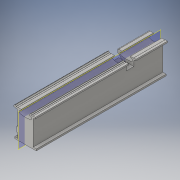
# Autodesk Inventor part: BED
Saved by Autodesk Inventor 2016 (Build 200138000, 138)
## iProperties
Created: 2017-02-14
Part Number: BED
Material: Generic
Document SubType Name: Modeling
Designer: M228540
Density: 1 g/cm^3
Appearance: Default
Author: M228540
Autodesk Inventor part; units mm, degrees
ref_plane "YZ Plane" through (0, 0, 0) normal (1, 0, 0) x (0, 1, 0)
ref_plane "XZ Plane" through (0, 0, 0) normal (0, 1, 0) x (-1, 0, 0)
ref_plane "XY Plane" through (0, 0, 0) normal (0, 0, 1) x (1, 0, 0)
sketch "Sketch1" plane through (0, 0, 0) normal (0, 0, 1) x (1, 0, 0)
  line L0 (11.5932, 5.302) -> (2.0669, 10.802)
  line L1 (11.5932, 5.302) -> (22.5932, 5.302) construction
  line L2 (2.0669, 10.802) -> (-7.9331, 10.802)
  line L3 (-7.9331, 10.802) -> (-7.9331, 22.502)
  line L4 (-7.9331, 22.502) -> (0.166, 32.1541)
  line L5 (0.166, 32.1541) -> (3.966, 32.1541)
  line L6 (3.966, 32.1541) -> (11.7797, 25.5977)
  line L7 (11.7797, 25.5977) -> (11.7797, 22.3977)
  line L8 (11.7797, 22.3977) -> (27.8797, 22.3977)
  line L9 (27.8797, 22.3977) -> (27.8797, 24.3977)
  line L10 (27.8797, 24.3977) -> (53.0797, 24.3977)
  line L11 (53.0797, 24.3977) -> (53.0797, 8.6977)
  line L12 (53.0797, 8.6977) -> (38.3797, 8.6977)
  line L13 (38.3797, 8.6977) -> (38.3797, 0.6977) construction
  line L14 (38.3797, 0.6977) -> (33.7609, 0.6977) construction
  line L15 (38.3797, 8.6977) -> (33.7609, 0.6977)
  line L16 (38.3797, 8.6977) -> (62.019, 8.6977) construction
  line L17 (33.7609, 0.6977) -> (33.7609, -3.3023) construction
  arc A0 (33.7609, 0.6977) -> (29.7609, -3.3023) centre (33.7609, -3.3023) ccw
  line L18 (29.7609, -3.3023) -> (29.7609, -65.3023)
  line L19 (29.7609, -65.3023) -> (29.7609, -269.3023)
  line L20 (-7.9331, 10.802) -> (84.2692, 10.802) construction
  line L21 (-100.1287, 11.7042) -> (-99.7212, 24.3977)
  line L22 (-99.7212, 24.3977) -> (-135.9212, 24.3977)
  line L23 (-99.7212, 24.3977) -> (-63.5212, 24.3977) construction
  line L24 (-135.9212, 24.3977) -> (-135.9212, 22.3977)
  line L25 (-135.9212, 22.3977) -> (-154.9212, 22.3977)
  line L26 (-154.9212, 22.3977) -> (-154.9212, 24.3977)
  line L27 (-154.9212, 24.3977) -> (-163.406, 34.5095)
  line L28 (-163.406, 34.5095) -> (-168.006, 34.5095)
  line L29 (-168.006, 34.5095) -> (-180.2627, 24.2249)
  line L30 (-180.2627, 24.2249) -> (-180.2627, 10.2249)
  line L31 (-180.2627, 10.2249) -> (-166.2627, 10.2249)
  line L32 (-166.2627, 10.2249) -> (-166.2627, 7.2249) construction
  line L33 (-166.2627, 7.2249) -> (-164.5307, 7.2249) construction
  line L34 (-166.2627, 10.2249) -> (-164.5307, 7.2249)
  line L35 (-166.2627, 10.2249) -> (-161.6857, 10.2249) construction
  line L36 (-164.5307, 7.2249) -> (-146.1307, 7.2249)
  line L37 (-146.1307, 7.2249) -> (-146.1307, -15.2751)
  line L38 (-146.1307, -15.2751) -> (-146.1307, -24.7751) construction
  arc A1 (-136.6307, -24.7751) -> (-146.1307, -15.2751) centre (-146.1307, -24.7751) ccw
  line L39 (-136.6307, -24.7751) -> (-136.6307, -160.7751)
  line L40 (-136.6307, -24.7751) -> (-0.6307, -24.7751) construction
  line L41 (-136.6307, -160.7751) -> (-149.6307, -160.7751)
  line L42 (-149.6307, -160.7751) -> (-149.6307, -216.2751)
  line L43 (-149.6307, -216.2751) -> (-136.6307, -216.2751)
  line L44 (-136.6307, -216.2751) -> (-136.6307, -269.3023)
  line L45 (-136.6307, -24.7751) -> (-146.1307, -24.7751) construction
  line L46 (29.7609, -3.3023) -> (33.7609, -3.3023) construction
  line L47 (-136.6307, -269.3023) -> (-171.6307, -269.3023)
  line L48 (-136.6307, -269.3023) -> (-101.6307, -269.3023) construction
  line L49 (-171.6307, -269.3023) -> (-171.6307, -287.3023)
  line L50 (29.7609, -269.3023) -> (64.7609, -269.3023)
  line L51 (29.7609, -269.3023) -> (64.7609, -269.3023) construction
  line L52 (64.7609, -269.3023) -> (64.7609, -287.3023)
  line L53 (64.7609, -287.3023) -> (-171.6307, -287.3023)
  line L54 (-100.1287, 11.7042) -> (-110.7287, 11.7042)
  line L55 (-100.1287, 11.7042) -> (-89.5287, 11.7042) construction
  line L56 (-110.7287, 11.7042) -> (-114.7287, 4.776)
  line L57 (-114.7287, 4.776) -> (-119.5691, 2.2026) construction
  line L58 (-119.5691, 2.2026) -> (-124.3726, -3.2958) construction
  line L59 (-124.3726, -3.2958) -> (-125.2569, -13.4593) construction
  line L60 (-125.2569, -13.4593) -> (-112.7287, -23.6091) construction
  line L61 (-112.7287, -23.6091) -> (-52.4666, -29.8459) construction
  line L62 (-52.4666, -29.8459) -> (0.1681, -24.7751) construction
  line L63 (0.1681, -24.7751) -> (13.3927, -18.0576) construction
  line L64 (13.3927, -18.0576) -> (19.8318, -6.9438) construction
  line L65 (19.8318, -6.9438) -> (14.7088, 3.5032) construction
  line L66 (14.7088, 3.5032) -> (11.5932, 5.302) construction
  spline S0 degree 4 poles (-114.7287, 4.776) (-119.5691, 2.2026) (-124.3726, -3.2958) (-125.2569, -13.4593) (-112.7287, -23.6091) (-52.4666, -29.8459) (0.1681, -24.7751) (13.3927, -18.0576) (19.8318, -6.9438) (14.7088, 3.5032) (11.5932, 5.302) knots 0 0 0 0 0 1 2 3 4 5 6 7 7 7 7 7
  point P0 (0, 0)
  dimension "d0" = 11
  dimension "d1" = 150
  dimension "d2" = 10
  dimension "d3" = 11.7
  dimension "d4" = 12.6
  dimension "d5" = 140
  dimension "d6" = 3.8
  dimension "d7" = 10.2
  dimension "d8" = 140
  dimension "d9" = 3.2
  dimension "d10" = 16.1
  dimension "d11" = 2
  dimension "d12" = 25.2
  dimension "d13" = 15.7
  dimension "d14" = 14.7
  dimension "d15" = 8
  dimension "d16" = 120
  dimension "d17" = 4
  dimension "d18" = 62
  dimension "d19" = 204
  dimension "d22" = 92.2
  dimension "d24" = 12.7
  dimension "d25" = 36.2
  dimension "d26" = 180
  dimension "d27" = 2
  dimension "d28" = 19
  dimension "d29" = 2
  dimension "d30" = 13.2
  dimension "d31" = 140
  dimension "d32" = 4.6
  dimension "d33" = 16
  dimension "d34" = 140
  dimension "d35" = 14
  dimension "d36" = 14
  dimension "d37" = 90
  dimension "d38" = 3
  dimension "d39" = 60
  dimension "d40" = 18.4
  dimension "d41" = 22.5
  dimension "d42" = 9.5
  dimension "d43" = 136
  dimension "d44" = 90
  dimension "d45" = 13
  dimension "d46" = 55.5
  dimension "d47" = 90
  dimension "d50" = 90
  dimension "d51" = 35
  dimension "d52" = 180
  dimension "d53" = 18
  dimension "d54" = 90
  dimension "d55" = 35
  dimension "d57" = 18
  dimension "d58" = 10.6
  dimension "d59" = 180
  dimension "d60" = 8
  dimension "d61" = 120
  dimension "d62" = 62
  constraints: 114 end point, 20 horizontal, 19 perpendicular, 6 equal length, 6 vertical, 4 point on circle, 4 point on line, 2 centre point, 2 coincident, 2 parallel, 1 collinear, 3 other
  measures "d0" distance of L0.start L0.end
  measures "d1" angle of L1 L0
  measures "d2" distance of L0.end L2.end
  measures "d3" distance of L2.end L3.end
  measures "d4" distance of L3.end L4.end
  measures "d5" angle of L3 L4
  measures "d6" distance of L4.end L5.end
  measures "d7" distance of L5.end L6.end
  measures "d8" angle of L5 L6
  measures "d9" distance of L6.end L7.end
  measures "d10" distance of L7.end L8.end
  measures "d11" distance of L8.end L9.end
  measures "d12" distance of L9.end L10.end
  measures "d13" distance of L10.end L11.end
  measures "d14" distance of L11.end L12.end
  measures "d15" distance of L12.end L13.end
  measures "d16" angle of L15 L16
  measures "d17" distance of L14.end L17.end
  measures "d18" distance of L18.start L18.end
  measures "d19" distance of L18.end L19.end
  measures "d22" distance of L2.end L21.start
  measures "d24" distance of L21.start L21.end
  measures "d25" distance of L21.end L22.end
  measures "d26" angle of L22 L23
  measures "d27" distance of L22.end L24.end
  measures "d28" distance of L24.end L25.end
  measures "d29" distance of L25.end L26.end
  measures "d30" distance of L26.end L27.end
  measures "d31" angle of L27 L26
  measures "d32" distance of L27.end L28.end
  measures "d33" distance of L28.end L29.end
  measures "d34" angle of L29 L28
  measures "d35" distance of L29.end L30.end
  measures "d36" distance of L30.end L31.end
  measures "d37" angle of L31 L30
  measures "d38" distance of L31.end L32.end
  measures "d39" angle of L34 L35
  measures "d40" distance of L33.end L36.end
  measures "d41" distance of L36.end L37.end
  measures "d42" distance of L37.end L38.end
  measures "d43" distance of L39.start L39.end
  measures "d44" angle of L39 L40
  measures "d45" distance of L39.end L41.end
  measures "d46" distance of L41.end L42.end
  measures "d47" angle of L42 L41
  measures "d50" angle of L43 L44
  measures "d51" distance of L44.end L47.end
  measures "d52" angle of L47 L48
  measures "d53" distance of L47.end L49.end
  measures "d54" angle of L49 L47
  measures "d55" distance of L19.end L50.end
  measures "d57" distance of L50.end L52.end
  measures "d58" distance of L21.start L54.end
  measures "d59" angle of L54 L55
  measures "d60" distance of L54.end L56.end
  measures "d61" angle of L56 L54
  measures "d62" distance from line of L5 L61.end
extrude "Extrusion1" add sketch "Sketch1" against normal blind 1420
chamfer "Chamfer1" distance 9 angle 45 2 edges at (-136.6307, -160.7751, -710) (-136.6307, -216.2751, -710)
ref_plane "Work Plane3" through (-63.5915, 24.2249, -1420) normal (-1, 0, 0) x (0, 0, 1)
sketch "Sketch2" plane through (-63.5915, 24.2249, -1420) normal (-1, 0, 0) x (0, 0, 1)
  line L0 (1420, 7.9293) -> (0, 7.9293) projected
  line L1 (400, 7.9293) -> (400, -79.7707)
  line L2 (400, -79.7707) -> (318, -79.7707)
  line L3 (318, -79.7707) -> (318, 139.9542)
  line L4 (1420, -27.5272) -> (0, -27.5272) projected
  line L5 (318, 139.9542) -> (400, 139.9542)
  line L6 (400, 139.9542) -> (400, 7.9293)
  line L7 (1420, -27.5272) -> (1420, -293.5272) projected
  point P0 (1420, -24.2249)
  dimension "d68" = 1020
  dimension "d69" = 82
  dimension "d70" = 87.7
  constraints: 10 end point, 4 perpendicular, 2 point on line, 1 vertical
  measures "d68" distance between parallel lines of L7 L1
  measures "d69" distance of L1.end L2.end
  measures "d70" distance between parallel lines of L2 L0
extrude "Extrusion2" cut sketch "Sketch2" along normal through all both and the other way through all
sketch "Sketch3" plane through (0, 0, -1420) normal (0, 0, -1) x (-1, 0, 0)
  line L0 (-11.7797, 22.3977) -> (13.8457, 22.3977)
  line L1 (13.8457, 22.3977) -> (13.8457, 35.6713)
  line L2 (13.8457, 35.6713) -> (-11.7797, 35.6713)
  line L3 (-11.7797, 25.5977) -> (-11.7797, 22.3977) projected
  line L4 (-11.7797, 35.6713) -> (-11.7797, 22.3977)
  point P0 (0, 0)
  constraints: 8 end point, 2 perpendicular, 1 collinear, 1 horizontal
extrude "Extrusion3" cut sketch "Sketch3" against normal up to surface (318 mm away)
sketch "Sketch4" plane through (0, 0, -1420) normal (0, 0, -1) x (-1, 0, 0)
  line L0 (164.5307, 7.2249) -> (146.1307, 7.2249) projected
  line L1 (146.1307, 7.2249) -> (146.1307, 38.8283)
  line L2 (146.1307, 38.8283) -> (190.7847, 38.8283)
  line L3 (190.7847, 38.8283) -> (190.7847, 7.2249)
  line L4 (190.7847, 7.2249) -> (146.1307, 7.2249)
  point P0 (0, 0)
  constraints: 8 end point, 2 perpendicular, 1 collinear, 1 vertical
extrude "Extrusion4" cut sketch "Sketch4" against normal up to surface (318 mm away)
sketch "Sketch5" plane through (0, 0, -1420) normal (0, 0, -1) x (-1, 0, 0)
  arc A0 (146.1307, -15.2751) -> (136.6307, -24.7751) centre (146.1307, -24.7751) ccw projected
  line L0 (141.489, -16.4863) -> (133.1179, -21.0771) construction
  line L1 (133.1179, -21.0771) -> (126.8668, -24.7751) construction
  line L2 (126.8668, -24.7751) -> (113.0712, -37.4594) construction
  line L3 (113.0712, -37.4594) -> (105.6307, -59.2751) construction
  line L4 (105.6307, -59.2751) -> (108.8696, -81.0371) construction
  line L5 (108.8696, -81.0371) -> (113.8852, -116.9822) construction
  line L6 (113.8852, -116.9822) -> (136.6307, -198.3023) construction
  spline S0 degree 4 poles (141.489, -16.4863) (133.1179, -21.0771) (126.8668, -24.7751) (113.0712, -37.4594) (105.6307, -59.2751) (108.8696, -81.0371) (113.8852, -116.9822) (136.6307, -198.3023) knots 1 1 1 1 1 2 3 4 5 5 5 5 5
  line L7 (171.6307, -269.3023) -> (136.6307, -269.3023) projected
  line L8 (136.6307, -151.7751) -> (136.6307, -24.7751) projected
  line L9 (136.6307, -269.3023) -> (136.6307, -225.2751) projected
  line L10 (136.6307, -198.3023) -> (136.6307, -225.2751)
  line L11 (136.6307, -225.2751) -> (162.5877, -225.2751)
  line L12 (162.5877, -225.2751) -> (148.4093, -16.0174)
  line L13 (148.4093, -16.0174) -> (141.489, -16.4863)
  point P0 (0, 0)
  dimension "d77" = 71
  dimension "d78" = 31
  dimension "d79" = 44
  constraints: 8 end point, 2 perpendicular, 1 collinear, 1 point on circle, 3 other
  measures "d77" distance from line of L7 L6.end
  measures "d78" distance from line of L8 L3.end
  measures "d79" vertical distance of A0.start L3.end
extrude "Extrusion5" cut sketch "Sketch5" against normal up to surface (318 mm away)
sketch "Sketch6" plane through (0, 0, -1420) normal (0, 0, -1) x (-1, 0, 0)
  line L0 (146.1307, 22.3977) -> (135.9212, 22.3977) projected
  line L1 (135.9212, 22.3977) -> (135.9212, 24.3977) projected
  line L2 (135.9212, 24.3977) -> (99.7212, 24.3977) projected
  line L3 (99.7212, 24.3977) -> (100.1287, 11.7042) projected
  line L4 (100.1287, 11.7042) -> (110.7287, 11.7042) projected
  line L5 (110.7287, 11.7042) -> (114.7287, 4.776) projected
  spline S0 degree 4 poles (114.7287, 4.776) (119.5691, 2.2026) (124.3726, -3.2958) (125.2569, -13.4593) (112.7287, -23.6091) (52.4666, -29.8459) (-0.1681, -24.7751) (-13.3927, -18.0576) (-19.8318, -6.9438) (-14.7088, 3.5032) (-11.5932, 5.302) knots 0 0 0 0 0 0.142857 0.285714 0.428571 0.571429 0.714286 0.857143 1 1 1 1 1 projected
  line L6 (146.1307, -15.2751) -> (146.1307, 22.3977) projected
  line L7 (-11.5932, 5.302) -> (-2.0669, 10.802) projected
  line L8 (-2.0669, 10.802) -> (7.9331, 10.802) projected
  line L9 (7.9331, 10.802) -> (7.9331, 22.3977) projected
  line L10 (7.9331, 22.3977) -> (-27.8797, 22.3977) projected
  line L11 (-27.8797, 24.3977) -> (-53.0797, 24.3977) projected
  line L12 (-27.8797, 22.3977) -> (-27.8797, 24.3977) projected
  line L13 (-53.0797, 24.3977) -> (-53.0797, 8.6977) projected
  line L14 (-53.0797, 8.6977) -> (-38.3797, 8.6977) projected
  line L15 (-38.3797, 8.6977) -> (-33.7609, 0.6977) projected
  arc A0 (-29.7609, -3.3023) -> (-33.7609, 0.6977) centre (-33.7609, -3.3023) ccw projected
  line L16 (-33.7609, 0.6977) -> (-15.3886, 0.6977)
  line L17 (120.2404, 0.6977) -> (146.1307, 0.6977)
  point P0 (0, 0)
  constraints: 4 end point, 2 perpendicular, 2 tangent, 1 point on line, 3 other
extrude "Extrusion6" add sketch "Sketch6" along normal blind 26
sketch "Sketch7" plane through (-146.1307, -15.2751, 0) normal (-1, 0, 0) x (0, 0, 1)
  circle A0 centre (-18.5, 9.5) radius 4
  circle A1 centre (-32.5, 9.5) radius 4
  line L0 (0, 22.5) -> (-1020, 22.5) projected
  line L1 (0, 0) -> (0, 22.5) projected
  point P0 (0, 15.2751)
  dimension "d85" = 13
  dimension "d86" = 18.5
  dimension "d87" = 14
  dimension "d88" = 8
  dimension "d89" = 8
  constraints: 2 centre point, 1 horizontal alignment
  measures "d85" distance from line of L0 A0.centre
  measures "d86" distance from line of L1 A0.centre
  measures "d87" distance of A0.centre A1.centre
  measures "d88" diameter of A0
  measures "d89" diameter of A1
extrude "Extrusion7" cut sketch "Sketch7" against normal blind 20
sketch "Sketch8" plane through (-149.6307, -216.2751, 0) normal (-1, 0, 0) x (0, 0, 1)
  circle A0 centre (-22.5, 38.5) radius 4
  circle A1 centre (-37.5, 38.5) radius 4
  line L0 (0, 0) -> (0, 55.5) projected
  circle A2 centre (-18.5, 210.5) radius 4 projected
  point P0 (0, 216.2751)
  dimension "d92" = 22.5
  dimension "d93" = 15
  dimension "d94" = 8
  dimension "d95" = 8
  dimension "d96" = 172
  constraints: 2 centre point, 1 horizontal alignment
  measures "d92" distance from line of L0 A0.centre
  measures "d93" distance of A0.centre A1.centre
  measures "d94" diameter of A0
  measures "d95" diameter of A1
  measures "d96" vertical distance of A2.centre A0.centre
extrude "Extrusion8" cut sketch "Sketch8" against normal blind 20 contours A0 | A1
body "Solid1"
